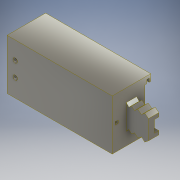
# Autodesk Inventor part: 装置容器
Saved by Autodesk Inventor 2018 (Build 220112000, 112)
## iProperties
Created: 2020-11-25
Part Number: 装置容器
Material: 银
Document SubType Name: Modeling
Designer: OHHHHHHHHHH
Density: 10.49 g/cm^3
Appearance: 银
Author: OHHHHHHHHHH
Autodesk Inventor part; units mm, degrees
ref_plane "YZ Plane" through (0, 0, 0) normal (1, 0, 0) x (0, 1, 0)
ref_plane "XZ Plane" through (0, 0, 0) normal (0, 1, 0) x (-1, 0, 0)
ref_plane "XY Plane" through (0, 0, 0) normal (0, 0, 1) x (1, 0, 0)
sketch "草图1" plane through (0, 0, 0) normal (0, 1, 0) x (-1, 0, 0)
  line L0 (0, 0) -> (0, -6.5)
  line L1 (0, 0) -> (15, 0)
  line L2 (0, 0) -> (0, -6.5)
  line L3 (0, -6.5) -> (2.5, -8.5)
  line L4 (2.5, -8.5) -> (4.6956, -6.5)
  line L5 (4.6956, -6.5) -> (7.1956, -8.5)
  line L6 (7.1956, -8.5) -> (9.3913, -6.5)
  line L7 (9.3913, -6.5) -> (11.4564, -8.1521)
  line L8 (11.4564, -8.1521) -> (13.2702, -6.5)
  line L9 (13.2702, -6.5) -> (15, -8.399)
  line L10 (15, 0) -> (82, 0)
  line L11 (82, 0) -> (82, -17)
  line L12 (82, -17) -> (15, -17)
  line L13 (15, -17) -> (15, -8.399)
  line L14 (15, -10) -> (15, -8.399)
  line L15 (15, -10) -> (15, -8.399)
  dimension "d1" = 6.5
  dimension "d2" = 15
  dimension "d3" = 99.01
  dimension "d4" = 67
  dimension "d6" = 17
  constraints: 32 end point, 6 parallel, 2 perpendicular, 1 coincident, 1 horizontal
  measures "d1" distance of L0.start L0.end
  measures "d2" horizontal distance of L0.end L9.end
  measures "d3" angle of L3 L4
  measures "d4" distance of L11.end L12.end
  measures "d6" distance between parallel lines of L12 L10
extrude "拉伸1" add sketch "草图1" along normal blind 26
sketch "草图2" plane through (-82, 0, -17) normal (-1, 0, 0) x (0, 0, 1)
  line L0 (4.4791, 22) -> (2, 22)
  line L1 (2, 22) -> (2, 2)
  line L2 (2, 2) -> (17, 2)
  line L3 (4.4791, 23.5) -> (2, 23.5)
  line L4 (2, 23.5) -> (2, 25)
  line L5 (2, 25) -> (4.4791, 25)
  line L6 (0, 0) -> (17, 0) projected
  line L7 (17, 0) -> (17, 26) projected
  line L8 (0, 26) -> (17, 26) projected
  line L9 (0, 0) -> (0, 26) projected
  line L10 (4.4791, 25) -> (4.4791, 26)
  line L11 (4.4791, 23.5) -> (4.4791, 22)
  line L12 (17, 0) -> (17, 26) projected
  line L13 (4.4791, 26) -> (17, 26)
  line L14 (17, 26) -> (17, 2)
  dimension "d9" = 20
  dimension "d11" = 1.5
  dimension "d12" = 1.5
  dimension "d13" = 15
  dimension "d14" = 2
  constraints: 20 end point, 5 perpendicular, 3 horizontal, 2 parallel, 2 point on line
  measures "d9" distance of L0.end L1.end
  measures "d11" distance between parallel lines of L0 L3
  measures "d12" distance between parallel lines of L3 L5
  measures "d13" distance of L1.end L2.end
  measures "d14" distance between parallel lines of L6 L2
extrude "拉伸2" cut sketch "草图2" against normal blind 65 contours L11 L3 L4 L5 L10 L8 L7 L2 L1 L0
sketch "草图3" plane through (-82, 0, -17) normal (-1, 0, 0) x (0, 0, 1)
  line L0 (0, 0) -> (0, 26) projected
  line L1 (0, 26) -> (17, 26)
  line L2 (17, 26) -> (17, 0)
  line L3 (17, 0) -> (0, 0)
  line L4 (0, 0) -> (0, 26)
  constraints: 8 end point, 2 parallel, 1 horizontal, 1 perpendicular
extrude "拉伸3" add sketch "草图3" along normal blind 4
mirror "镜像1" about plane through (-82, 0, 0) normal (0, 0, 1) of "拉伸1", "拉伸2", "拉伸3"
sketch "草图4" plane through (0, 26, 0) normal (0, 1, 0) x (1, 0, 0)
  line L0 (-15, -17) -> (-86, -17) projected
  line L1 (-15, -8.399) -> (-15, -17) projected
  line L2 (-13.2702, -6.5) -> (-15, -8.399) projected
  line L3 (-11.4564, -8.1521) -> (-13.2702, -6.5) projected
  line L4 (-9.3913, -6.5) -> (-11.4564, -8.1521) projected
  line L5 (-7.1956, -8.5) -> (-9.3913, -6.5) projected
  line L6 (-4.6956, -6.5) -> (-7.1956, -8.5) projected
  line L7 (-2.5, -8.5) -> (-4.6956, -6.5) projected
  line L8 (0, -6.5) -> (-2.5, -8.5) projected
  line L9 (0, 6.5) -> (0, -6.5) projected
  line L10 (0, 6.5) -> (-2.5, 8.5) projected
  line L11 (-2.5, 8.5) -> (-4.6956, 6.5) projected
  line L12 (-4.6956, 6.5) -> (-7.1956, 8.5) projected
  line L13 (-7.1956, 8.5) -> (-9.3913, 6.5) projected
  line L14 (-9.3913, 6.5) -> (-11.4564, 8.1521) projected
  line L15 (-11.4564, 8.1521) -> (-13.2702, 6.5) projected
  line L16 (-13.2702, 6.5) -> (-15, 8.399) projected
  line L17 (-15, 8.399) -> (-15, 17) projected
  line L18 (-15, 17) -> (-86, 17) projected
  line L19 (-86, 17) -> (-86, -17) projected
  line L20 (-82, 12.5209) -> (-82, -12.5209) projected
  line L21 (-82, 12.5209) -> (-17, 12.5209) projected
  line L22 (-17, 12.5209) -> (-17, -12.5209) projected
  line L23 (-17, -12.5209) -> (-82, -12.5209) projected
  line L24 (-15, -8.399) -> (-15, 8.399)
  point P0 (0, 0)
  constraints: 2 end point, 1 collinear
extrude "拉伸4" cut sketch "草图4" against normal blind 9.5 contours L24 L16 L15 L14 L13 L12 L11 L10 L9 L8 L7 L6 L5 L4 L3 L2
ref_plane "工作平面1" through (0, 13, 0) normal (0, 1, 0) x (1, 0, 0)
mirror "镜像2" about plane through (0, 13, 0) normal (0, 1, 0) of "拉伸4"
sketch "草图5" plane through (-15, 0, -17) normal (1, 0, 0) x (0, 0, -1)
  line L0 (-32, 23.5) -> (-32, 25) projected
  line L1 (-4.4791, 23.5) -> (-2, 23.5) projected
  line L2 (-32, 25) -> (-2, 25)
  line L3 (-2, 25) -> (-2, 23.5)
  line L4 (-2, 23.5) -> (-32, 23.5)
  line L5 (-32, 23.5) -> (-32, 25)
  line L6 (-29.5209, 25) -> (-29.5209, 26) projected
  line L7 (-4.4791, 25) -> (-4.4791, 26) projected
  line L8 (-29.5209, 25) -> (-4.4791, 25)
  line L9 (-4.4791, 25) -> (-4.4791, 26)
  line L10 (-4.4791, 26) -> (-29.5209, 26)
  line L11 (-29.5209, 26) -> (-29.5209, 25)
  line L12 (-32, 22) -> (-29.5209, 22) projected
  line L13 (-29.5209, 22) -> (-4.4791, 22)
  line L14 (-4.4791, 22) -> (-4.4791, 23.5)
  line L15 (-4.4791, 23.5) -> (-29.5209, 23.5)
  line L16 (-29.5209, 23.5) -> (-29.5209, 22)
  point P0 (-17, 0)
  constraints: 24 end point, 6 parallel, 3 horizontal, 3 perpendicular, 2 point on line
extrude "拉伸5" cut sketch "草图5" against normal up to surface (2 mm away) from surface at 0
sketch "草图6" plane through (0, 16.5, 6.5) normal (1, 0, 0) x (0, 0, -1)
  line L0 (0, -7) -> (13, -7) projected
  line L1 (13, -7) -> (13, 0) projected
  line L2 (13, 0) -> (0, 0) projected
  line L3 (0, -7) -> (0, 0) projected
  line L4 (0, -3) -> (13, -3) projected
  line L5 (2.5, 0) -> (10.5, 0)
  line L6 (10.5, 0) -> (10.5, -3)
  line L7 (10.5, -3) -> (2.5, -3)
  line L8 (2.5, -3) -> (2.5, 0)
  line L9 (0, -7) -> (0, 0) projected
  line L10 (6.5, -3) -> (6.5, 0)
  line L11 (13, 0) -> (0, 0) projected
  dimension "d23" = 8
  dimension "d24" = 3
  constraints: 10 end point, 2 midpoint, 1 collinear, 1 horizontal, 1 parallel, 1 perpendicular, 1 other
  measures "d23" distance of L5.start L5.end
  measures "d24" distance of L5.end L6.end
extrude "拉伸6" cut sketch "草图6" against normal blind 68.25 contours L8 L2 L10 L4 | L4 L10 L2 L6
sketch "草图7" plane through (0, 0, 0) normal (0, -1, 0) x (1, 0, 0)
  line L0 (-82, 15) -> (-82, -15) projected
  line L1 (-82, -15) -> (-17, -15) projected
  line L2 (-82, 15) -> (-17, 15) projected
  circle A0 centre (-80.5, -5) radius 1.5
  circle A1 centre (-80.5, 5) radius 1.5
  line L3 (-103.2, 0) -> (17.2, 0) projected
  point P0 (0, 0)
  dimension "d27" = 3
  dimension "d28" = 3
  dimension "d29" = 10
  dimension "d30" = 1.5
  constraints: 2 centre point, 1 symmetric about line
  measures "d27" diameter of A0
  measures "d28" diameter of A1
  measures "d29" distance of A1.centre A0.centre
  measures "d30" distance from line of L0 A0.centre
extrude "拉伸7" cut sketch "草图7" against normal blind 9.25
sketch "草图8" plane through (-15, 0, -17) normal (1, 0, 0) x (0, 0, -1)
  line L0 (-17.9721, 4) -> (-15.9721, 4)
  line L1 (-15.9721, 4) -> (-15.9721, 2)
  line L2 (-15.9721, 2) -> (-17.9721, 2)
  line L3 (-17.9721, 2) -> (-17.9721, 4)
  line L4 (-16.9721, 7.1271) -> (-16.9721, -1.5009)
  line L5 (0, 0) -> (-34, 0) projected
  point P0 (-17, 0)
  dimension "d33" = 2
  dimension "d34" = 2
  dimension "d35" = 2
  constraints: 10 end point, 2 parallel, 1 horizontal, 1 perpendicular, 1 vertical, 1 other
  measures "d33" distance of L0.start L0.end
  measures "d34" distance of L0.end L1.end
  measures "d35" distance between parallel lines of L5 L2
extrude "拉伸8" cut sketch "草图8" against normal blind 5
